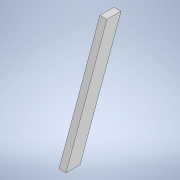
# Autodesk Inventor part: Support Bracket 1
Saved by Autodesk Inventor 2020 (Build 240168000, 168)
## iProperties
Created: 2021-01-18
Part Number: Support Bracket 1
Material: Generic
Document SubType Name: Modeling
Designer: magda
Density: 1 g/cm^3
Appearance: Default
Author: magda
Autodesk Inventor part; units mm, degrees
ref_plane "YZ Plane" through (0, 0, 0) normal (1, 0, 0) x (0, 1, 0)
ref_plane "XZ Plane" through (0, 0, 0) normal (0, 1, 0) x (-1, 0, 0)
ref_plane "XY Plane" through (0, 0, 0) normal (0, 0, 1) x (1, 0, 0)
sketch "Sketch1" plane through (0, 0, 0) normal (1, 0, 0) x (0, 1, 0)
  line L0 (0, 0) -> (0, -25.4)
  line L1 (203.2, -73.9588) -> (203.2, -99.3588)
  line L2 (0, 0) -> (203.2, -73.9588)
  line L3 (0, -25.4) -> (203.2, -99.3588)
  line L4 (0, 0) -> (68.675, 0)
  dimension "d0" = 25.4
  dimension "d5" = 25.4
  dimension "d6" = 20
  dimension "d7" = 203.2
  constraints: 10 end point, 2 vertical, 1 horizontal
  measures "d0" distance of L1.start L1.end
  measures "d5" distance of L0.start L0.end
  measures "d6" angle of L2 L4
  measures "d7" distance between parallel lines of L1 L0
extrude "Extrusion1" add sketch "Sketch1" along normal blind 12.7
body "Solid1"
